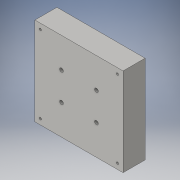
# Autodesk Inventor part: Adapter_V_522_and_Sutter_V4
Saved by Autodesk Inventor 2016 (Build 200138000, 138)
## iProperties
Created: 2018-07-19
Part Number: Adapter_V_522_and_Sutter_V4
Material: Generic
Document SubType Name: Modeling
Designer: FiolkaLab
Density: 1 g/cm^3
Appearance: Default
Author: FiolkaLab
Autodesk Inventor part; units mm, degrees
ref_plane "YZ Plane" through (0, 0, 0) normal (1, 0, 0) x (0, 1, 0)
ref_plane "XZ Plane" through (0, 0, 0) normal (0, 1, 0) x (-1, 0, 0)
ref_plane "XY Plane" through (0, 0, 0) normal (0, 0, 1) x (1, 0, 0)
sketch "Sketch2" plane through (0, 0, 0) normal (0, 0, 1) x (1, 0, 0)
  line L0 (0, 0) -> (80, 0)
  line L1 (80, 0) -> (80, 80)
  line L2 (80, 80) -> (0, 80)
  line L3 (0, 80) -> (0, 0)
  dimension "d0" = 80
  dimension "d1" = 80
  constraints: 8 end point, 2 parallel, 1 horizontal, 1 perpendicular
  measures "d0" distance of L2.end L1.end
  measures "d1" distance of L0.end L1.end
extrude "Extrusion1" add sketch "Sketch2" along normal blind 20
sketch "Sketch3" plane through (0, 0, 20) normal (0, 0, 1) x (1, 0, 0)
  circle A0 centre (5, 75) radius 1.25
  line L0 (0, 80) -> (0, 0) projected
  line L1 (80, 80) -> (0, 80) projected
  circle A1 centre (5, 5) radius 1.25
  line L2 (0, 0) -> (80, 0) projected
  circle A2 centre (75, 75) radius 1.25
  line L3 (80, 0) -> (80, 80) projected
  circle A3 centre (75, 5) radius 1.25
  dimension "d4" = 2.5
  dimension "d5" = 5
  dimension "d6" = 5
  dimension "d7" = 5
  dimension "d8" = 5
  dimension "d9" = 2.5
  dimension "d10" = 5
  dimension "d11" = 5
  dimension "d12" = 2.5
  dimension "d39" = 5
  dimension "d40" = 5
  constraints: 4 centre point
  measures "d4" diameter of A0
  measures "d5" distance from line of L0 A0.centre
  measures "d6" distance from line of L1 A0.centre
  measures "d7" distance from line of L0 A1.centre
  measures "d8" distance from line of L2 A1.centre
  measures "d9" diameter of A2
  measures "d10" distance from line of L3 A2.centre
  measures "d11" distance from line of L1 A2.centre
  measures "d12" diameter of A3
  measures "d39" distance from line of L3 A3.centre
  measures "d40" distance from line of L2 A3.centre
hole "Hole1" at (5, 75, 20) at (75, 75, 20) at (75, 5, 20) at (5, 5, 20) direction (0, 0, -1) diameter 2.013 end through all thread size "M2.5x0.45" class "6H" standard "ANSI Metric M Profile"
sketch "Sketch4" plane through (0, 0, 0) normal (0, 0, -1) x (-1, 0, 0)
  circle A0 centre (-55.875, 52.7) radius 1.5
  circle A1 centre (-24.125, 52.7) radius 1.5
  circle A2 centre (-24.125, 27.3) radius 1.5
  circle A3 centre (-55.875, 27.3) radius 1.5
  line L0 (-80, 0) -> (-80, 80) projected
  line L1 (-80, 80) -> (0, 80) projected
  point P0 (0, 0)
  dimension "d20" = 24.125
  dimension "d21" = 24.125
  dimension "d22" = 27.3
  dimension "d23" = 27.3
  dimension "d24" = 31.75
  dimension "d25" = 31.75
  dimension "d26" = 25.4
  dimension "d27" = 25.4
  dimension "d28" = 3
  dimension "d29" = 3
  dimension "d30" = 3
  dimension "d31" = 3
  constraints: 4 centre point
  measures "d20" distance from line of A0.centre L0
  measures "d21" distance from line of L0 A3.centre
  measures "d22" distance from line of L1 A0.centre
  measures "d23" distance from line of L1 A1.centre
  measures "d24" distance of A1.centre A0.centre
  measures "d25" distance of A2.centre A3.centre
  measures "d26" distance of A1.centre A2.centre
  measures "d27" distance of A0.centre A3.centre
  measures "d28" diameter of A0
  measures "d29" diameter of A1
  measures "d30" diameter of A3
  measures "d31" diameter of A2
hole "Hole2" at (55.875, 52.7, 0) at (24.125, 52.7, 0) at (24.125, 27.3, 0) at (55.875, 27.3, 0) direction (0, 0, 1) diameter 3.4 end through all counterbore diameter 6 counterbore depth 5 clearance for "Hex Head Cap Screw DIN EN 24017" size "M3" standard "DIN"
equation "\"d21\" = d20"
equation "\"d25\" = d24"
equation "\"d29\" = d28"
equation "\"d30\" = d28"
equation "\"d31\" = d29"
body "Solid1"
